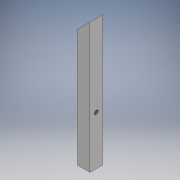
# Autodesk Inventor part: Part2
Saved by Autodesk Inventor 2018 (Build 220112000, 112)
## iProperties
Created: 2017-09-07
Part Number: Part2
Material: 一般
Document SubType Name: Modeling
Designer: Kosei
Density: 1 g/cm^3
Appearance: 既定
Author: Kosei
Autodesk Inventor part; units mm, degrees
ref_plane "YZ Plane" through (0, 0, 0) normal (1, 0, 0) x (0, 1, 0)
ref_plane "XZ Plane" through (0, 0, 0) normal (0, 1, 0) x (-1, 0, 0)
ref_plane "XY Plane" through (0, 0, 0) normal (0, 0, 1) x (1, 0, 0)
sketch "スケッチ1" plane through (0, 0, 0) normal (0, 0, 1) x (1, 0, 0)
  line L0 (16, 16) -> (-16, 16)
  line L1 (-16, 16) -> (-16, -16)
  line L2 (-16, -16) -> (16, -16)
  line L3 (16, -16) -> (16, 16)
  line L4 (14.4, 14.4) -> (-14.4, 14.4)
  line L5 (-14.4, 14.4) -> (-14.4, -14.4)
  line L6 (-14.4, -14.4) -> (14.4, -14.4)
  line L7 (14.4, -14.4) -> (14.4, 14.4)
  point P0 (0, 0)
  dimension "d6" = 32
  dimension "d7" = 32
  dimension "d8" = 1.6
  dimension "d24" = 16
  dimension "d26" = 16
  constraints: 16 end point, 4 parallel, 2 perpendicular, 1 horizontal, 3 other
  measures "d6" distance of L2.end L1.end
  measures "d7" distance of L1.end L0.end
  measures "d8" distance between parallel lines of L3 L7
  measures "d24" distance from line of point (0, 0) L1
  measures "d26" distance from line of point (0, 0) L0
extrude "押し出し3" add sketch "スケッチ1" along normal blind 330
sketch "スケッチ7" plane through (16, -16, 0) normal (1, 0, 0) x (0, 0, -1)
  line L0 (0, 0) -> (0, 32) projected
  line L1 (0, 0) -> (-330, 0) projected
  point P0 (0, 16)
  point P1 (-124, 16)
  dimension "d15" = 124
  dimension "d16" = 16
  measures "d15" distance from line of L0 point (-124, 16)
  measures "d16" distance from line of L1 point (-124, 16)
hole "穴1" at (16, 0, 124) direction (-1, 0, 0) diameter 10.5 end through all
chamfer "面取り2" distance 32 angle 45 1 edges at (-16, 0, 330)
